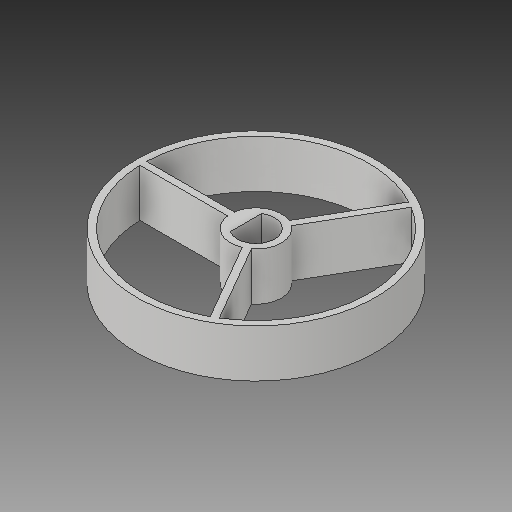
# Autodesk Inventor part: Wheel
Saved by Autodesk Inventor 2018 (Build 220112000, 112)
## iProperties
Created: 2018-01-30
Part Number: Wheel
Material: Generic
Document SubType Name: Modeling
Designer: alber
Density: 1 g/cm^3
Appearance: Default
Mass: 3.3947 g
Surface Area: 53.1421 cm^2
Volume: 3.3947 cm^3
Author: alber
Autodesk Inventor part; units mm, degrees
ref_plane "YZ Plane" through (0, 0, 0) normal (1, 0, 0) x (0, 1, 0)
ref_plane "XZ Plane" through (0, 0, 0) normal (0, 1, 0) x (-1, 0, 0)
ref_plane "XY Plane" through (0, 0, 0) normal (0, 0, 1) x (1, 0, 0)
sketch "Sketch1" plane through (0, 0, 0) normal (0, 1, 0) x (-1, 0, 0)
  circle A0 centre (0, 0) radius 25
  dimension "d0" = 50
  constraints: 1 centre point, 1 coincident
  measures "d0" diameter of A0
extrude "Extrusion1" add sketch "Sketch1" along normal blind 10
sketch "Sketch2" plane through (0, 10, 0) normal (0, 1, 0) x (1, 0, 0)
  arc A0 (-2.1, -3.2863) -> (-2.1, 3.2863) centre (0, 0) ccw
  line L0 (-2.1, -3.2863) -> (-2.1, 3.2863)
  dimension "d3" = 7.8
  dimension "d4" = 2.1
  constraints: 2 end point, 2 point on circle, 1 centre point, 1 coincident, 1 vertical
  measures "d3" diameter of A0
  measures "d4" distance from line of point (0, 0) L0
extrude "Extrusion2" cut sketch "Sketch2" against normal up to surface (10 mm away)
sketch "Sketch3" plane through (0, 10, 0) normal (0, 1, 0) x (1, 0, 0)
  line L0 (-2.1, -3.2863) -> (-2.1, 3.2863) projected
  arc A0 (-2.1, -3.2863) -> (-2.1, 3.2863) centre (0, 0) ccw projected
  circle A1 centre (0, 0) radius 25 projected
  line L1 (-23.5896, -0.7) -> (-5.2536, -0.7)
  line L2 (-23.5896, 0.7) -> (-5.2536, 0.7)
  line L3 (11.1886, 20.7792) -> (2.0206, 4.8997)
  line L4 (12.401, 20.0792) -> (3.233, 4.1997)
  line L5 (12.401, -20.0792) -> (3.233, -4.1997)
  line L6 (11.1886, -20.7792) -> (2.0206, -4.8997)
  arc A2 (3.233, -4.1997) -> (3.233, 4.1997) centre (0, 0) ccw
  arc A3 (12.401, -20.0792) -> (12.401, 20.0792) centre (0, 0) ccw
  arc A4 (2.0206, 4.8997) -> (-5.2536, 0.7) centre (0, 0) ccw
  arc A5 (-5.2536, -0.7) -> (2.0206, -4.8997) centre (0, 0) ccw
  arc A6 (11.1886, 20.7792) -> (-23.5896, 0.7) centre (0, 0) ccw
  arc A7 (-23.5896, -0.7) -> (11.1886, -20.7792) centre (0, 0) ccw
  dimension "d9" = 1.4
  dimension "d12" = 360
  constraints: 12 end point, 12 point on circle, 6 centre point, 2 parallel, 1 coincident, 1 horizontal, 19 other
  measures "d9" distance between parallel lines of L2 L1
extrude "Extrusion3" cut sketch "Sketch3" against normal through all contours L1 A5 L6 A7 | A6 L3 A4 L2 | A3 L5 A2 L4
body "Solid1"
